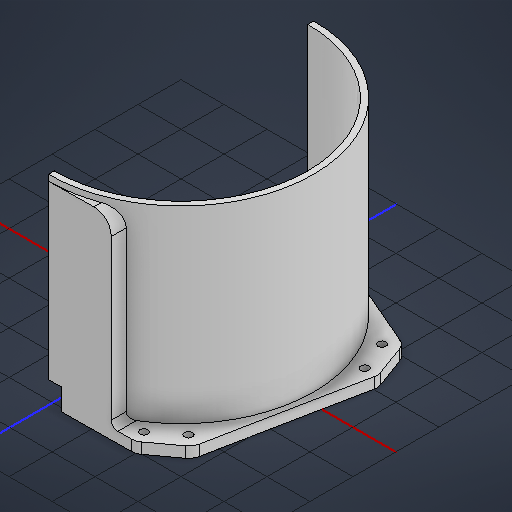
# Autodesk Inventor part: 000.010.003 - Кожух
Saved by Autodesk Inventor 2025 (Build 290162000, 162)
## iProperties
Created: 2024-08-25
Part Number: 000.010.003 - Кожух
Material: Типовые
Document SubType Name: Modeling
Designer: IvanPetrov
Density: 1 g/cm^3
Appearance: По умолчанию
Author: IvanPetrov
Autodesk Inventor part; units mm, degrees
ref_plane "YZ Plane" through (0, 0, 0) normal (1, 0, 0) x (0, 1, 0)
ref_plane "XZ Plane" through (0, 0, 0) normal (0, 1, 0) x (-1, 0, 0)
ref_plane "XY Plane" through (0, 0, 0) normal (0, 0, 1) x (1, 0, 0)
sketch "Эскиз1" plane through (0, 0, 0) normal (0, 1, 0) x (-1, 0, 0)
  arc A0 (0, 61.75) -> (0, -61.75) centre (0, 0) ccw
  arc A1 (0, 59) -> (0, -59) centre (0, 0) ccw
  line L0 (0, 61.75) -> (0, 59)
  line L1 (0, -59) -> (0, -61.75)
  dimension "d0" = 123.5
  dimension "d1" = 118
  constraints: 4 end point, 4 point on circle, 2 centre point, 2 coincident, 2 point on line, 1 vertical
  measures "d0" diameter of A0
  measures "d1" diameter of A1
extrude "Выдавливание1" add sketch "Эскиз1" along normal blind 92.75
sketch "Эскиз3" plane through (0, 0, 0) normal (0, -1, 0) x (1, 0, 0)
  circle A0 centre (64.0005, -21.501) radius 1.85 projected
  circle A1 centre (58.3434, -35.1577) radius 1.85 projected
  circle A2 centre (58.3434, -35.1577) radius 6.3677
  arc A3 (0, -61.75) -> (0, 61.75) centre (0, 0) ccw projected
  circle A4 centre (64.0005, -21.501) radius 5.7656
  line L0 (64.3207, -37.353) -> (69.4126, -23.4886)
  line L1 (69.5587, -19.9687) -> (59.5292, 16.4113)
  line L2 (60.8642, -41.0052) -> (24.4455, -56.7052)
  constraints: 8 tangent, 6 end point, 6 point on circle, 2 centre point, 2 coincident
extrude "Выдавливание3" add sketch "Эскиз3" against normal blind 5
pattern_circular "Круговой массив1" count 2 over 74 about axis through (0, 0, 0) along (0, -1, 0) of "Выдавливание3"
fillet "Сопряжение1" radius 12874.75 1 edges at (60.6901, 2.5, 12.2006)
sketch "Эскиз4" plane through (38.3681, 0, 61.36) normal (0.0102493, 0, 0.9999475) x (0.9999475, 0, -0.0102493)
  line L0 (-38.37, 0) -> (-32.37, 0)
  line L1 (-38.37, 0) -> (-38.37, 92.75) projected
  line L2 (-38.37, 0) -> (-32.37, 0)
  line L3 (-32.37, 0) -> (-32.37, 10)
  line L4 (-32.37, 10) -> (-38.37, 10)
  line L5 (-38.37, 10) -> (-38.37, 0)
  point P0 (-37.7372, 0)
  point P1 (-32.37, 0)
  dimension "d15" = 6
  dimension "d16" = 10
  constraints: 10 end point, 2 horizontal, 2 parallel, 1 perpendicular
  measures "d15" distance of L4.end L3.end
  measures "d16" distance of L3.end L2.end
extrude "Выдавливание4" cut sketch "Эскиз4" against normal blind 5
sketch "Эскиз6" plane through (0, 5, 0) normal (0, 1, 0) x (1, 0, 0)
  line L0 (29, -62.4615) -> (29, -61.456)
  line L1 (5.9997, -61.6917) -> (38.3681, -61.36) projected
  line L2 (0, -59) -> (0, -61.75) projected
  arc A0 (5.9973, -61.4581) -> (24.4455, 56.7052) centre (0, 0) ccw construction
  arc A1 (0, -61.75) -> (0, 61.75) centre (0, 0) ccw projected
  line L3 (5.9973, -61.4581) -> (5.9997, -61.6917) projected
  line L4 (29, -61.456) -> (29, -54.5166)
  point P0 (0, -60.375)
  dimension "d19" = 29
  constraints: 4 end point, 2 vertical, 1 midpoint, 1 point on circle, 1 point on line
  measures "d19" distance from line of point (0, -60.375) L0
extrude "Выдавливание5" add sketch "Эскиз6" along normal blind 85
fillet "Сопряжение2" radius 8 1 edges at (29, 90, 57.9863)
sketch "Эскиз7" plane through (5.969, 0, 58.6973) normal (-0.9999475, 0, 0.0102493) x (0.0102493, 0, 0.9999475)
  line L0 (2.7609, 10) -> (0, 10) projected
  line L1 (2.7609, 10) -> (2.9946, 10)
  line L2 (2.9946, 90) -> (2.9946, 0) projected
  line L3 (2.7609, 90) -> (2.9946, 90) projected
  line L4 (2.7609, 10) -> (2.7609, 90) projected
  point P0 (-58.7554, 0)
  constraints: 2 end point, 1 horizontal, 1 point on line
extrude "Выдавливание6" add sketch "Эскиз7" along normal up to surface surface through (0, 0, 59) normal (-1, 0, 0)
fillet "Сопряжение3" radius 3 1 edges at (29, 5, 57.9863)
